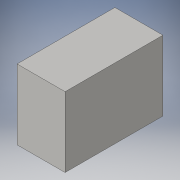
# Autodesk Inventor part: AmplifierBlock2
Saved by Autodesk Inventor 2016 (Build 200138000, 138)
## iProperties
Created: 2016-08-31
Part Number: AmplifierBlock2
Material: Generic
Document SubType Name: Modeling
Designer: jfixelle
Density: 1 g/cm^3
Appearance: Default
Author: jfixelle
Autodesk Inventor part; units mm, degrees
ref_plane "YZ Plane" through (0, 0, 0) normal (1, 0, 0) x (0, 1, 0)
ref_plane "XZ Plane" through (0, 0, 0) normal (0, 1, 0) x (-1, 0, 0)
ref_plane "XY Plane" through (0, 0, 0) normal (0, 0, 1) x (1, 0, 0)
sketch "Sketch1" plane through (0, 0, 0) normal (0, 1, 0) x (-1, 0, 0)
  line L0 (3.2862, 6.5013) -> (-3.5718, 6.5013)
  line L1 (-3.5718, 6.5013) -> (-3.5718, -7.4687)
  line L2 (-3.5718, -7.4687) -> (3.2862, -7.4687)
  line L3 (3.2862, -7.4687) -> (3.2862, 6.5013)
  point P0 (0, 0)
  dimension "d0" = 13.97
  dimension "d1" = 6.858
  constraints: 8 end point, 2 parallel, 1 horizontal, 1 perpendicular
  measures "d0" distance of L2.end L0.start
  measures "d1" distance of L1.end L2.end
extrude "Extrusion1" add sketch "Sketch1" along normal blind 10
body "Solid1"
